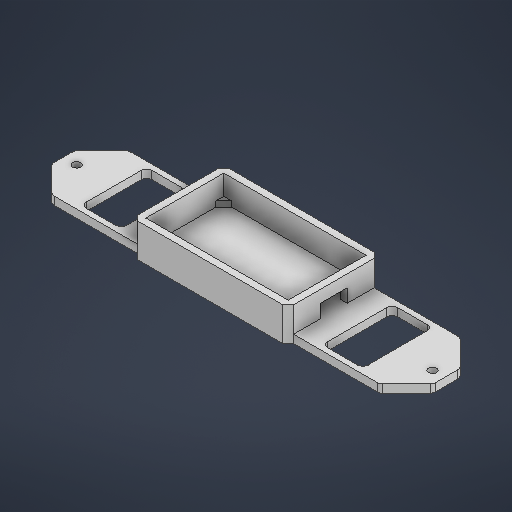
# Autodesk Inventor part: espbase
Saved by Autodesk Inventor 2026 (Build 300175050, 175E)
## iProperties
Created: 2025-04-01
Part Number: espbase
Material: Genérico
Document SubType Name: Modeling
Designer: Ian
Density: 1 g/cm^3
Appearance: Padrão
Author: Ian
Autodesk Inventor part; units mm, degrees
ref_plane "YZ Plane" through (0, 0, 0) normal (1, 0, 0) x (0, 1, 0)
ref_plane "XZ Plane" through (0, 0, 0) normal (0, 1, 0) x (-1, 0, 0)
ref_plane "XY Plane" through (0, 0, 0) normal (0, 0, 1) x (1, 0, 0)
sketch "Esboço1" plane through (0, 0, 0) normal (0, 1, 0) x (-1, 0, 0)
  line L0 (-29, 17) -> (29, 17)
  line L1 (29, 17) -> (29, -17)
  line L2 (29, -17) -> (-29, -17)
  line L3 (-29, -17) -> (-29, 17)
  line L4 (-29, 17) -> (29, -17) construction
  line L5 (29, 17) -> (-29, -17) construction
  point P0 (0, 0)
  point P1 (0.0565, -0.0161)
  dimension "d0" = 58
  dimension "d1" = 34
  constraints: 12 end point, 2 midpoint, 2 parallel, 1 horizontal, 1 perpendicular
  measures "d0" distance of L1.end L2.end
  measures "d1" distance of L0.end L1.end
extrude "Extrusão1" add sketch "Esboço1" along normal blind 3
sketch "Esboço2" plane through (0, 3, 0) normal (0, 1, 0) x (1, 0, 0)
  line L0 (26.5, -14.5) -> (-26.5, -14.5)
  line L1 (-26.5, -14.5) -> (-26.5, 14.5)
  line L2 (-26.5, 14.5) -> (26.5, 14.5)
  line L3 (26.5, 14.5) -> (26.5, -14.5)
  line L4 (26.5, -14.5) -> (-26.5, 14.5) construction
  line L5 (-26.5, -14.5) -> (26.5, 14.5) construction
  line L6 (29, 17) -> (-29, 17) projected
  line L7 (29, -17) -> (-29, -17)
  line L8 (-29, -17) -> (-29, 17)
  line L9 (-29, 17) -> (29, 17)
  line L10 (29, 17) -> (29, -17)
  line L11 (29, -17) -> (-29, 17) construction
  line L12 (-29, -17) -> (29, 17) construction
  point P0 (0, 0)
  dimension "d4" = 53
  dimension "d5" = 29
  constraints: 24 end point, 4 midpoint, 4 parallel, 2 horizontal, 2 perpendicular
  measures "d4" distance of L1.end L2.end
  measures "d5" distance of L0.end L1.end
extrude "Extrusão2" add sketch "Esboço2" along normal blind 9.5
sketch "Esboço3" plane through (0, 3, 0) normal (0, 1, 0) x (1, 0, 0)
  line L0 (-26.5, 14.5) -> (26.5, 14.5) projected
  line L1 (-26.5, -14.5) -> (-26.5, 14.5) projected
  line L2 (26.5, 14.5) -> (26.5, -14.5) projected
  line L3 (26.5, -14.5) -> (-26.5, -14.5) projected
  line L4 (-23.5, -14.5) -> (-26.5, -14.5)
  line L5 (-26.5, -14.5) -> (-26.5, -11.5)
  line L6 (-26.5, -11.5) -> (-23.5, -11.5)
  line L7 (-23.5, -11.5) -> (-23.5, -14.5)
  line L8 (-23.5, -14.5) -> (-26.5, -11.5) construction
  line L9 (-26.5, -14.5) -> (-23.5, -11.5) construction
  line L10 (-23.5, 11.5) -> (-26.5, 11.5)
  line L11 (-26.5, 11.5) -> (-26.5, 14.5)
  line L12 (-26.5, 14.5) -> (-23.5, 14.5)
  line L13 (-23.5, 14.5) -> (-23.5, 11.5)
  line L14 (-23.5, 11.5) -> (-26.5, 14.5) construction
  line L15 (-26.5, 11.5) -> (-23.5, 14.5) construction
  line L16 (26.5, -14.5) -> (23.5, -14.5)
  line L17 (23.5, -14.5) -> (23.5, -11.5)
  line L18 (23.5, -11.5) -> (26.5, -11.5)
  line L19 (26.5, -11.5) -> (26.5, -14.5)
  line L20 (26.5, -14.5) -> (23.5, -11.5) construction
  line L21 (23.5, -14.5) -> (26.5, -11.5) construction
  line L22 (26.5, 11.5) -> (23.5, 11.5)
  line L23 (23.5, 11.5) -> (23.5, 14.5)
  line L24 (23.5, 14.5) -> (26.5, 14.5)
  line L25 (26.5, 14.5) -> (26.5, 11.5)
  line L26 (26.5, 11.5) -> (23.5, 14.5) construction
  line L27 (23.5, 11.5) -> (26.5, 14.5) construction
  point P0 (0, 0)
  point P1 (-13.75, -16.75)
  point P2 (-13.75, 16.75)
  point P3 (13.75, 16.75)
  point P4 (13.75, -16.75)
  point P5 (-26.5, -13)
  dimension "d66" = 3
  dimension "d67" = 3
  dimension "d68" = 3
  dimension "d69" = 3
  dimension "d70" = 3
  dimension "d71" = 3
  dimension "d72" = 3
  dimension "d73" = 3
  dimension "d74" = 0
  dimension "d75" = 0
  dimension "d76" = 0
  dimension "d77" = 0
  dimension "d78" = 0
  dimension "d79" = 0
  dimension "d80" = 0
  dimension "d81" = 0
  constraints: 48 end point, 8 parallel, 4 horizontal, 4 perpendicular, 1 midpoint, 2 other
  measures "d66" distance of L5.end L6.end
  measures "d67" distance of L4.end L5.end
  measures "d68" distance of L11.end L12.end
  measures "d69" distance of L10.end L11.end
  measures "d70" distance of L17.end L18.end
  measures "d71" distance of L16.end L17.end
  measures "d72" distance of L23.end L24.end
  measures "d73" distance of L22.end L23.end
  measures "d74" distance between parallel lines of L3 L4
  measures "d76" horizontal extent of L11
  measures "d77" distance between parallel lines of L0 L12
  measures "d78" horizontal extent of L19
  measures "d79" distance between parallel lines of L3 L16
  measures "d80" horizontal extent of L25
  measures "d81" distance between parallel lines of L0 L24
extrude "Extrusão3" add sketch "Esboço3" along normal blind 2 contours L0 L13 L10 L1 | L0 L2 L22 L23 | L6 L7 L3 L1 | L2 L3 L17 L18
chamfer "Chanfro1" distance 2 angle 45 4 edges at (29, 6.25, 17) (-29, 6.25, 17) (-29, 6.25, -17) (29, 6.25, -17)
sketch "Esboço7" plane through (29, 0, 15) normal (1, 0, 0) x (0, 0, -1)
  line L0 (30, 0) -> (0, 0) projected
  line L1 (0, 0) -> (30, 0)
  line L2 (30, 0) -> (30, 3)
  line L3 (30, 3) -> (0, 3)
  line L4 (0, 3) -> (0, 0)
  line L5 (30, 12.5) -> (30, 0) projected
  line L6 (0, 0) -> (0, 12.5) projected
  point P0 (15, 0)
  point P1 (15, 0)
  point P2 (15, 3)
  dimension "d36" = 3
  dimension "d42" = 0
  dimension "d43" = 0
  constraints: 8 end point, 2 midpoint, 2 parallel, 1 horizontal, 1 perpendicular, 1 point on line
  measures "d36" distance of L2.end L1.end
  measures "d42" horizontal distance of point (15, 0) point (15, 3)
  measures "d43" distance between parallel lines of L6 L4
extrude "Extrusão6" add sketch "Esboço7" along normal blind 42.04
sketch "Esboço9" plane through (-29, 0, -15) normal (-1, 0, 0) x (0, 0, 1)
  line L0 (30, 12.5) -> (30, 0) projected
  line L1 (1.5, 0) -> (30, 0)
  line L2 (30, 0) -> (30, 3)
  line L3 (30, 3) -> (1.5, 3)
  line L4 (1.5, 3) -> (1.5, 0)
  point P0 (15, 0)
  dimension "d59" = 3
  constraints: 8 end point, 2 parallel, 1 horizontal, 1 perpendicular, 1 point on line
  measures "d59" distance of L2.end L1.end
extrude "Extrusão8" add sketch "Esboço9" along normal blind 42.04
sketch "Esboço8" plane through (29, 3, 15) normal (0, 1, 0) x (1, 0, 0)
  circle A0 centre (37.5465, 14.25) radius 1.5
  line L0 (0, 0) -> (0, 30) projected
  line L1 (23.7495, 2) -> (8.7495, 2)
  line L2 (8.7495, 2) -> (8.7495, 28)
  line L3 (8.7495, 28) -> (23.7495, 28)
  line L4 (23.7495, 28) -> (23.7495, 2)
  line L5 (0, 0) -> (42.04, 0) projected
  line L6 (0, 30) -> (42.04, 30) projected
  line L7 (-2, 32) -> (-56, 32) projected
  line L8 (-56, -2) -> (-2, -2) projected
  circle A1 centre (-95.0465, 14.25) radius 1.5
  line L9 (-81.2495, 2) -> (-66.2495, 2)
  line L10 (-66.2495, 2) -> (-66.2495, 26.5)
  line L11 (-66.2495, 26.5) -> (-81.2495, 26.5)
  line L12 (-81.2495, 26.5) -> (-81.2495, 2)
  point P0 (-29, 15)
  point P1 (23.7495, 15)
  point P2 (-81.2495, 14.25)
  dimension "d44" = 3
  dimension "d47" = 13.797
  dimension "d53" = 2
  dimension "d54" = 2
  dimension "d55" = 15
  constraints: 16 end point, 2 centre point, 2 parallel, 1 horizontal, 1 midpoint, 1 perpendicular
  measures "d44" diameter of A0
  measures "d47" horizontal distance of point (23.749, 15) A0.centre
  measures "d53" distance between parallel lines of L5 L1
  measures "d54" distance between parallel lines of L6 L3
  measures "d55" distance between parallel lines of L2 L4
extrude "Extrusão7" cut sketch "Esboço8" against normal blind 42.04
chamfer "Chanfro2" distance 10 angle 45 4 edges at (71.04, 1.5, -15) (71.04, 1.5, 15) (-71.04, 1.5, -13.5) (-71.04, 1.5, 15)
sketch "Esboço10" plane through (29, 12.5, 15) normal (1, 0, 0) x (0, 0, -1)
  line L0 (0, -9.5) -> (30, -9.5) projected
  line L1 (30, 0) -> (30, -9.5) projected
  line L2 (0, 0) -> (30, 0) projected
  line L3 (0, -9.5) -> (0, 0) projected
  line L4 (10, -12.5) -> (10, -9.5) projected
  line L5 (10, -12.5) -> (20, -12.5) projected
  line L6 (20, -9.5) -> (20, -12.5) projected
  line L7 (20, -9.5) -> (10, -9.5) projected
  line L8 (5, -9.5) -> (20, -9.5)
  line L9 (20, -9.5) -> (20, -4.5)
  line L10 (20, -4.5) -> (10, -4.5)
  line L11 (10, -4.5) -> (10, -9.5)
  point P0 (15, -12.5)
  point P1 (20, -9.5)
  point P2 (15, 0)
  point P3 (15, -4.5)
  dimension "d82" = 10
  dimension "d83" = 0
  dimension "d84" = 4.5
  dimension "d85" = 0
  dimension "d86" = 5
  constraints: 8 end point, 2 midpoint, 2 parallel, 1 horizontal, 1 perpendicular
  measures "d82" distance of L9.end L10.end
  measures "d83" horizontal distance of point (15, 0) point (15, -4.5)
  measures "d84" distance between parallel lines of L2 L10
  measures "d85" distance between parallel lines of L0 L8
  measures "d86" distance of L8.end L9.end
extrude "Extrusão9" cut sketch "Esboço10" against normal blind 10 contours L11 L10 L9 L0
chamfer "Chanfro3" distance 3 angle 45 4 edges at (-23.5, 4, 11.5) (-23.5, 4, -11.5) (23.5, 4, -11.5) (23.5, 4, 11.5)
fillet "Arredondamento1" radius 2 8 edges at (-37.2495, 1.5, -11.5) (-37.2495, 1.5, 13) (-52.2495, 1.5, -11.5) (-52.2495, 1.5, 13) (37.7495, 1.5, -13) (37.7495, 1.5, 13) (52.7495, 1.5, -13) (52.7495, 1.5, 13)
fillet "Arredondamento2" radius 2 8 edges at (71.04, 1.5, -5) (71.04, 1.5, 5) (61.04, 1.5, -15) (61.04, 1.5, 15) (-61.04, 1.5, -13.5) (-71.04, 1.5, -3.5) (-71.04, 1.5, 5) (-61.04, 1.5, 15)
